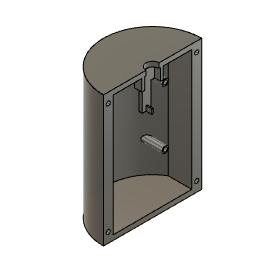
Shell4L v1 (Autodesk Fusion 360 design; units mm, degrees)
Autodesk Fusion 360 part; units mm, degrees
sketch "Sketch1" plane through (0, 0, 0) normal (0, 1, 0) x (1, 0, 0)
  circle A0 centre (0, 0) radius 38.1
  dimension "d1" = 76.2
  constraint coincident A0.centre origin
  measures "d1" diameter of A0
extrude "Extrude1" add sketch "Sketch1" against normal blind 101.6
sketch "Sketch2" plane through (0, 0, 0) normal (0, 1, 0) x (1, 0, 0)
  circle A0 centre (0, 0) radius 35.56
  dimension "d4" = 71.12
  constraint coincident A0.centre origin
  measures "d4" diameter of A0
extrude "Extrude2" cut sketch "Sketch2" against normal blind 154.94
sketch "Sketch3" plane through (0, 0, 0) normal (0, 1, 0) x (1, 0, 0)
  line L0 (0, 38.1) -> (0, -38.1)
  circle A0 centre (0, 0) radius 35.56
  circle A1 centre (0, 0) radius 38.1
  constraint vertical L0
  constraint coincident A0.centre A1.centre
  constraint concentric A0 A1
  constraint coincident L0.start A1
extrude "Extrude3" cut sketch "Sketch3" against normal blind 116.84 contours L0 A0 A1 picked at (3.4943, -37.0034)
sketch "Sketch4" plane through (0, 0, 0) normal (1, 0, 0) x (0, 0, -1)
  line L0 (35.56, -101.6) -> (38.1, -101.6)
  line L1 (38.1, -101.6) -> (38.1, 0)
  line L2 (38.1, 0) -> (35.56, 0)
  line L3 (35.56, 0) -> (35.56, -101.6)
  line L4 (38.1, 0) -> (30.48, 0)
  line L5 (30.48, 0) -> (30.48, -101.6)
  line L6 (30.48, -101.6) -> (38.1, -101.6)
  line L7 (38.1, -101.6) -> (38.1, 0)
  line L8 (-38.1, 0) -> (-30.48, 0)
  line L9 (-30.48, 0) -> (-30.48, -101.6)
  line L10 (-30.48, -101.6) -> (-38.1, -101.6)
  line L11 (-38.1, -101.6) -> (-38.1, 0)
  constraint horizontal L4
  constraint vertical L5
  constraint horizontal L6
  constraint vertical L7
  constraint coincident L1.end L2.start
  constraint horizontal L8
  constraint vertical L9
  constraint horizontal L10
  constraint vertical L11
extrude "Extrude4" add sketch "Sketch4" against normal blind 55.88 contours L3 L4 L5 L6 | L8 L9 L10 L11
sketch "Sketch5" plane through (0, 0, 0) normal (0, 1, 0) x (-1, 0, 0)
  line L0 (0, -30.48) -> (0, -38.1)
  arc A0 (0, -38.1) -> (13.6783, -35.56) centre (0, 0) ccw
  line L1 (13.6783, -35.56) -> (55.88, -35.56)
  line L2 (55.88, -35.56) -> (55.88, -30.48)
  line L3 (55.88, -30.48) -> (22.86, -30.48)
  arc A1 (22.86, -30.48) -> (22.86, 30.48) centre (0, 0) ccw
  line L4 (22.86, 30.48) -> (55.88, 30.48)
  line L5 (55.88, 30.48) -> (55.88, 38.1)
  line L6 (55.88, 38.1) -> (0, 38.1)
  line L7 (0, 38.1) -> (0, 30.48)
  line L8 (0, 30.48) -> (18.3162, 30.48)
  arc A2 (18.3162, -30.48) -> (18.3162, 30.48) centre (0, 0) ccw
  line L9 (18.3162, -30.48) -> (0, -30.48)
  circle A3 centre (0, 0) radius 38.1
  circle A4 centre (0, 0) radius 71.8421
  constraint concentric A0 A3
  constraint concentric A0 A4
extrude "Extrude5" cut sketch "Sketch5" against normal blind 121.92 contours L1 L2 L3 A3 | L4 L5 L6 A3 | A4
sketch "Sketch6" plane through (0, 0, 0) normal (1, 0, 0) x (0, 0, -1)
  line L0 (35.56, -101.6) -> (38.1, -101.6)
  line L1 (38.1, -101.6) -> (38.1, 0)
  line L2 (38.1, 0) -> (30.48, 0)
  line L3 (30.48, 0) -> (30.48, -101.6)
  line L4 (30.48, -101.6) -> (35.56, -101.6)
  line L5 (-30.48, 0) -> (30.48, 0)
  circle A0 centre (22.6462, -28.194) radius 2.5
  circle A1 centre (-22.5658, -28.194) radius 2.5
  circle A2 centre (22.6462, -73.406) radius 2.5
  circle A3 centre (-22.5658, -73.406) radius 2.5
  dimension "d22" = 5
  dimension "d23" = 5
  dimension "d24" = 5
  dimension "d25" = 5
  constraint horizontal L5
  measures "d22" diameter of A0
  measures "d23" diameter of A1
  measures "d24" diameter of A2
  measures "d25" diameter of A3
extrude "Extrude6" add sketch "Sketch6" against normal blind 33.02 contours A0 | A1 | A2 | A3
sketch "Sketch7" plane through (0, 0, 0) normal (0, 1, 0) x (-1, 0, 0)
  arc A0 (0, -38.1) -> (0, 38.1) centre (0, 0) ccw
  line L0 (0, 38.1) -> (0, 30.48)
  line L1 (0, 30.48) -> (18.3162, 30.48)
  arc A1 (18.3162, -30.48) -> (18.3162, 30.48) centre (0, 0) ccw
  line L2 (18.3162, -30.48) -> (0, -30.48)
  line L3 (0, -30.48) -> (0, -38.1)
  circle A2 centre (0, 0) radius 38.1
  circle A3 centre (0, 0) radius 58.6405
  constraint concentric A0 A2
  constraint coincident A0.start A2
  constraint concentric A2 A3
extrude "Extrude7" cut sketch "Sketch7" against normal blind 109.22
sketch "Sketch8" plane through (0, 0, 0) normal (1, 0, 0) x (0, 0, -1)
  circle A0 centre (-22.5658, -28.194) radius 2.5
  circle A1 centre (-22.5658, -28.194) radius 1.625
  line L0 (-38.1, 0) -> (-30.48, 0)
  line L1 (-30.48, -101.6) -> (-38.1, -101.6)
  line L2 (-30.48, -93.98) -> (-38.1, -93.98)
  circle A2 centre (-34.29, -93.98) radius 1.625
  line L3 (-38.1, -7.62) -> (-30.48, -7.62)
  circle A3 centre (-34.29, -7.62) radius 1.625
  dimension "d30" = 3.25
  dimension "d33" = 7.62
  dimension "d34" = 3.25
  dimension "d35" = 7.62
  dimension "d36" = 3.25
  constraint concentric A0 A1
  constraint horizontal L0
  constraint horizontal L1
  constraint midpoint L2 A2.centre
  constraint midpoint L3 A3.centre
  measures "d30" diameter of A1
  measures "d33" distance of L1
  measures "d34" diameter of A2
  measures "d35" distance of L0
  measures "d36" diameter of A3
extrude "Extrude8" cut sketch "Sketch8" against normal blind 4 contours L2 A2 | L2 A2 | L3 A3 | L3 A3
sketch "Sketch9" plane through (0, 0, 0) normal (1, 0, 0) x (0, 0, -1)
  line L0 (35.56, -101.6) -> (38.1, -101.6)
  line L1 (38.1, -101.6) -> (38.1, 0)
  line L2 (38.1, 0) -> (30.48, 0)
  line L3 (30.48, -101.6) -> (35.56, -101.6)
  line L4 (30.48, 0) -> (38.1, 0)
  line L5 (38.1, -101.6) -> (30.48, -101.6)
  circle A0 centre (34.29, -93.98) radius 1.625
  circle A1 centre (34.29, -7.62) radius 1.625
  dimension "d42" = 3.25
  dimension "d43" = 3.25
  constraint horizontal L4
  constraint horizontal L5
  constraint coincident L0.end L1.start
  constraint coincident L2.end L4.start
  measures "d42" diameter of A0
  measures "d43" diameter of A1
extrude "Extrude9" cut sketch "Sketch9" against normal blind 4
sketch "Sketch10" plane through (0, 0, 0) normal (1, 0, 0) x (0, 0, -1)
  circle A0 centre (-34.29, -7.62) radius 1.625
  circle A1 centre (-34.29, -93.98) radius 1.625
  line L0 (-38.1, -101.6) -> (-35.56, -101.6)
  line L1 (-35.56, -101.6) -> (-30.48, -101.6)
  line L2 (-30.48, -101.6) -> (-30.48, 0)
  line L3 (-30.48, 0) -> (-38.1, 0)
  line L4 (-38.1, 0) -> (-38.1, -101.6)
  line L5 (-30.48, 0) -> (30.48, 0)
  line L6 (30.48, 0) -> (30.48, -2.54)
  line L7 (30.48, -2.54) -> (-30.48, -2.54)
  line L8 (-30.48, -2.54) -> (-30.48, 0)
  constraint horizontal L5
  constraint vertical L6
  constraint horizontal L7
  constraint vertical L8
  constraint coincident L2.end L3.start
extrude "Extrude10" add sketch "Sketch10" against normal blind 35.56 contours L2 L5 L6 L7 L8
sketch "Sketch11" plane through (0, 0, 0) normal (0, 1, 0) x (-1, 0, 0)
  line L0 (0, 38.1) -> (0, -38.1)
  arc A0 (0, -38.1) -> (22.86, -30.48) centre (0, 0) ccw
  line L1 (22.86, -30.48) -> (35.56, -30.48)
  line L2 (35.56, -30.48) -> (35.56, -13.6783)
  arc A1 (35.56, -13.6783) -> (35.56, 13.6783) centre (0, 0) ccw
  line L3 (35.56, 13.6783) -> (35.56, 30.48)
  line L4 (35.56, 30.48) -> (22.86, 30.48)
  arc A2 (22.86, 30.48) -> (0, 38.1) centre (0, 0) ccw
  circle A3 centre (0, 0) radius 38.1
  circle A4 centre (0, 0) radius 51.0534
  constraint coincident A0.centre A1.centre
extrude "Extrude11" cut sketch "Sketch11" against normal blind 20.32 contours L3 L4 A3 | L1 L2 A3
sketch "Sketch12" plane through (0, 0, 0) normal (1, 0, 0) x (0, 0, -1)
  circle A0 centre (-34.29, -93.98) radius 1.625
  circle A1 centre (-34.29, -7.62) radius 1.625
  circle A2 centre (34.29, -93.98) radius 1.625
  circle A3 centre (34.29, -7.62) radius 1.625
  line L0 (35.56, -101.6) -> (38.1, -101.6)
  line L1 (38.1, -101.6) -> (38.1, 0)
  line L2 (38.1, 0) -> (-38.1, 0)
  line L3 (-38.1, 0) -> (-38.1, -101.6)
  line L4 (-38.1, -101.6) -> (-35.56, -101.6)
  line L5 (-35.56, -101.6) -> (-30.48, -101.6)
  line L6 (-30.48, -101.6) -> (-30.48, -2.54)
  line L7 (-30.48, -2.54) -> (30.48, -2.54)
  line L8 (30.48, -2.54) -> (30.48, -101.6)
  line L9 (30.48, -101.6) -> (35.56, -101.6)
  line L10 (-30.48, -101.6) -> (30.48, -101.6)
  line L11 (30.48, -101.6) -> (30.48, -99.06)
  line L12 (30.48, -99.06) -> (-30.48, -99.06)
  line L13 (-30.48, -99.06) -> (-30.48, -101.6)
  constraint horizontal L10
  constraint vertical L11
  constraint horizontal L12
  constraint vertical L13
  constraint coincident L8 L11.end
  constraint coincident L5.end L6.start
extrude "Extrude12" add sketch "Sketch12" against normal blind 38.1 contours L6 L8 L10 L11 L12 L13
sketch "Sketch13" plane through (0, -101.6, 0) normal (0, -1, 0) x (1, 0, 0)
  arc A0 (-22.86, -30.48) -> (0, -38.1) centre (0, 0) ccw
  line L0 (0, -38.1) -> (0, -35.56)
  line L1 (0, -35.56) -> (0, -30.48)
  line L2 (0, -30.48) -> (0, 35.56)
  line L3 (0, 35.56) -> (0, 38.1)
  arc A1 (0, 38.1) -> (-22.86, 30.48) centre (0, 0) ccw
  line L4 (-22.86, 30.48) -> (-38.1, 30.48)
  line L5 (-38.1, 30.48) -> (-38.1, -30.48)
  line L6 (-38.1, -30.48) -> (-22.86, -30.48)
  circle A2 centre (0, 0) radius 38.1
  circle A3 centre (0, 0) radius 53.4004
  constraint coincident A0.centre A1.centre
  constraint coincident L3.end A2
  constraint concentric A2 A3
extrude "Extrude13" cut sketch "Sketch13" against normal blind 43.18 contours L5 L6 A2 | L4 L5 A2
extrude "Extrude14" add 1 faces at (-11.8533, -99.06, 0) along direction (0, 1, 0) blind 2.54
extrude "Extrude15" cut 1 faces at (-11.8533, -96.52, 0) along direction (0, -1, 0) blind 1.27
extrude "Extrude16" add 1 faces at (-11.8533, -2.54, 0) along direction (0, -1, 0) blind 1.27
sketch "Sketch14" plane through (0, -3.81, 0) normal (0, -1, 0) x (1, 0, 0)
  arc A0 (-18.3162, 30.48) -> (-18.3162, -30.48) centre (0, 0) ccw
  line L0 (-18.3162, -30.48) -> (0, -30.48)
  line L1 (0, -30.48) -> (0, 30.48)
  line L2 (0, 30.48) -> (-18.3162, 30.48)
  line L3 (-4.572, 0) -> (-4.572, -6.096)
  line L4 (-4.572, -6.096) -> (0, -6.096)
  line L5 (0, -6.096) -> (0, 0)
  line L6 (-4.572, 0) -> (-4.572, 6.096)
  line L7 (-4.572, 6.096) -> (0, 6.096)
  line L8 (0, 6.096) -> (0, 0)
  line L9 (0.9906, 7.0866) -> (0.9906, 0)
  line L10 (0.9906, -7.0866) -> (0.9906, 0)
  line L11 (-5.5626, -7.0866) -> (0.9906, -7.0866)
  line L12 (-5.5626, 0) -> (-5.5626, -7.0866)
  line L13 (-5.5626, 0) -> (-5.5626, 7.0866)
  line L14 (-5.5626, 7.0866) -> (0.9906, 7.0866)
  dimension "d60" = 6.096
  dimension "d61" = 4.572
  dimension "d62" = 6.096
  dimension "d63" = 4.572
  dimension "d64" = -0.9906
  constraint vertical L3
  constraint horizontal L4
  constraint vertical L5
  constraint coincident A0.centre L5.end
  constraint vertical L6
  constraint horizontal L7
  constraint vertical L8
  measures "d60" distance of A0.centre L4.end
  measures "d61" distance of A0.centre L3.start
  measures "d62" distance of A0.centre L7.end
  measures "d63" distance of A0.centre L3.start
extrude "Extrude17" add sketch "Sketch14" along normal blind 9.144 contours L1 L3 L4 L6 L7 L11 L12 L13 L14
sketch "Sketch15" plane through (0, -12.954, 0) normal (0, -1, 0) x (1, 0, 0)
  line L0 (-5.5626, 7.0866) -> (-5.5626, -7.0866)
  line L1 (-5.5626, -7.0866) -> (0, -7.0866)
  line L2 (0, -7.0866) -> (0, -6.096)
  line L3 (0, -6.096) -> (-4.572, -6.096)
  line L4 (-4.572, -6.096) -> (-4.572, 6.096)
  line L5 (-4.572, 6.096) -> (0, 6.096)
  line L6 (0, 6.096) -> (0, 7.0866)
  line L7 (0, 7.0866) -> (-5.5626, 7.0866)
  line L8 (-5.5626, 3.3686) -> (-4.572, 3.3686)
  line L9 (-4.572, 3.3686) -> (-4.572, -3.3301)
  line L10 (-4.572, -3.3301) -> (-5.5626, -3.3301)
  line L11 (-5.5626, -3.3301) -> (-5.5626, 3.3686)
  constraint horizontal L8
  constraint vertical L9
  constraint horizontal L10
  constraint vertical L11
  constraint coincident L4 L9.end
  constraint coincident L0 L8.start
extrude "Extrude18" add sketch "Sketch15" along normal blind 15.24 contours L0 L4 L8 L9 L10 L11
extrude "Extrude19" add 1 faces at (-5.2324, -28.194, -1.0972) along direction (0, -1, 0) blind 1.27
sketch "Sketch16" plane through (-4.572, 0, 0) normal (1, 0, 0) x (0, 0, -1)
  line L0 (6.096, -3.81) -> (-6.096, -3.81)
  line L1 (-6.096, -3.81) -> (-6.096, -12.954)
  line L2 (-6.096, -12.954) -> (-3.3686, -12.954)
  line L3 (-3.3686, -12.954) -> (-3.3686, -29.464)
  line L4 (-3.3686, -29.464) -> (3.3301, -29.464)
  line L5 (3.3301, -29.464) -> (3.3301, -12.954)
  line L6 (3.3301, -12.954) -> (6.096, -12.954)
  line L7 (6.096, -12.954) -> (6.096, -3.81)
  line L8 (-3.3686, -29.464) -> (3.3301, -29.464)
  line L9 (3.3301, -29.464) -> (3.3301, -28.194)
  line L10 (3.3301, -28.194) -> (-3.3686, -28.194)
  line L11 (-3.3686, -28.194) -> (-3.3686, -29.464)
  line L12 (-0.0192, -28.194) -> (-0.5296, -28.194)
  line L13 (-0.5296, -28.194) -> (-0.5296, -29.464)
  line L14 (-0.5296, -29.464) -> (-0.0192, -29.464)
  line L15 (-0.0192, -28.194) -> (0.4841, -28.194)
  line L16 (0.4841, -28.194) -> (0.4841, -29.464)
  line L17 (0.4841, -29.464) -> (-0.0192, -29.464)
  dimension "d71" = 1.27
  constraint horizontal L8
  constraint vertical L9
  constraint horizontal L10
  constraint vertical L11
  constraint coincident L3.end L4.start
  constraint horizontal L12
  constraint vertical L13
  constraint horizontal L14
  constraint coincident L4 L13.end
  constraint midpoint L10 L12.start
  constraint horizontal L15
  constraint vertical L16
  constraint horizontal L17
  constraint coincident L8 L16.end
  measures "d71" distance of L3.end L10.end
extrude "Extrude20" add sketch "Sketch16" along normal blind 4.572 contours L4 L8 L10 L12 L13 L14 L15 L16 L17
sketch "Sketch17" plane through (0, 0, 0) normal (0, 1, 0) x (-1, 0, 0)
  arc A0 (0, -38.1) -> (0, 38.1) centre (0, 0) ccw
  line L0 (0, 38.1) -> (0, -38.1)
  circle A1 centre (0, 0) radius 5.08
  constraint coincident A0.centre A1.centre
extrude "Extrude21" cut sketch "Sketch17" against normal blind 3.81 contours L0 A1 picked at (2.4602, 1.1933)
extrude "Extrude22" cut 4 faces at (0, -29.025, 21.7947) (0, -28.5556, -23.397) (0, -73.0757, -24.573) (0, -73.0757, 20.639) along direction (-1, 0, 0) blind 7.62
extrude "Extrude23" cut 4 faces at (-7.62, -29.025, 21.7947) (-7.62, -28.5556, -23.397) (-7.62, -73.0757, -24.573) (-7.62, -73.0757, 20.639) along direction (-1, 0, 0) blind 5.08
sketch "Sketch18" plane through (-12.7, 0, 0) normal (1, 0, 0) x (0, 0, -1)
  circle A0 centre (-22.5658, -28.194) radius 2.5
  circle A1 centre (-22.5658, -28.194) radius 1.625
  dimension "d80" = 3.25
  constraint concentric A0 A1
  measures "d80" diameter of A1
extrude "Extrude24" cut sketch "Sketch18" against normal blind 4 contours A1
sketch "Sketch19" plane through (-12.7, 0, 0) normal (1, 0, 0) x (0, 0, -1)
  circle A0 centre (22.6462, -28.194) radius 2.5
  circle A1 centre (22.6462, -28.194) radius 1.625
  dimension "d83" = 3.25
  constraint concentric A0 A1
  measures "d83" diameter of A1
extrude "Extrude25" cut sketch "Sketch19" against normal blind 4 contours A1
sketch "Sketch20" plane through (-12.7, 0, 0) normal (1, 0, 0) x (0, 0, -1)
  circle A0 centre (22.6462, -73.406) radius 2.5
  circle A1 centre (22.6462, -73.406) radius 1.625
  dimension "d86" = 3.25
  constraint concentric A0 A1
  measures "d86" diameter of A1
extrude "Extrude26" cut sketch "Sketch20" against normal blind 4 contours A1
sketch "Sketch21" plane through (-12.7, 0, 0) normal (1, 0, 0) x (0, 0, -1)
  circle A0 centre (-22.5658, -73.406) radius 2.5
  circle A1 centre (-22.5658, -73.406) radius 1.625
  dimension "d89" = 3.25
  constraint concentric A0 A1
  measures "d89" diameter of A1
extrude "Extrude27" cut sketch "Sketch21" against normal blind 4 contours A1
extrude "Extrude28" add 1 faces at (-1.8542, -6.858, 7.0866) along direction (0, 0, 1) blind 1.27
extrude "Extrude29" add 1 faces at (-1.8542, -6.858, -7.0866) along direction (0, 0, -1) blind 1.27
extrude "Extrude30" add 1 faces at (-4.572, -18.034, -0.1485) along direction (-1, 0, 0) blind 2.54
extrude "Extrude31" add 1 faces at (-6.0791, -28.194, -0.1462) along direction (0, -1, 0) blind 1.27
extrude "Extrude32" add 1 faces at (-6.2653, -29.464, -0.1485) along direction (0, -1, 0) blind 2.54
sketch "Sketch22" plane through (0, -101.6, 0) normal (0, -1, 0) x (1, 0, 0)
  arc A0 (-22.86, 30.48) -> (-22.86, -30.48) centre (0, 0) ccw
  arc A1 (-22.86, -30.48) -> (0, -38.1) centre (0, 0) ccw
  line L0 (0, -38.1) -> (0, -35.56)
  line L1 (0, -35.56) -> (0, -30.48)
  line L2 (0, -30.48) -> (0, 35.56)
  line L3 (0, 35.56) -> (0, 38.1)
  arc A2 (0, 38.1) -> (-22.86, 30.48) centre (0, 0) ccw
